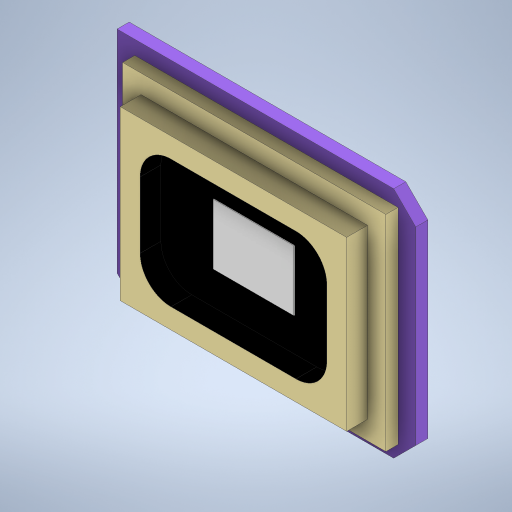
# Autodesk Inventor part: DLP
Saved by Autodesk Inventor 2024 (Build 280153000, 153)
## iProperties
Created: 2024-09-23
Part Number: DLP
Material: Generic
Document SubType Name: Modeling
Designer: PC
Density: 1 g/cm^3
Appearance: Default
Author: PC
Autodesk Inventor part; units mm, degrees
ref_plane "YZ Plane" through (0, 0, 0) normal (1, 0, 0) x (0, 1, 0)
ref_plane "XZ Plane" through (0, 0, 0) normal (0, 1, 0) x (-1, 0, 0)
ref_plane "XY Plane" through (0, 0, 0) normal (0, 0, 1) x (1, 0, 0)
sketch "Sketch1" plane through (0, 0, 0) normal (0, 0, 1) x (1, 0, 0)
  line L0 (3, 0) -> (40.64, 0)
  line L1 (37.64, 31.75) -> (0, 31.75)
  line L2 (0, 31.75) -> (0, 3)
  line L3 (37.64, 31.75) -> (40.64, 28.75)
  line L4 (3, 0) -> (0, 3)
  line L5 (40.64, 3) -> (37.64, 0)
  line L6 (40.64, 28.75) -> (40.64, 3)
  point P0 (0, 0)
  dimension "d4" = 3
  dimension "d5" = 45
  dimension "d6" = 45
  dimension "d7" = 3
  dimension "d8" = 31.75
  dimension "d9" = 40.64
  dimension "d10" = 3
  constraints: 14 end point, 10 coincident, 3 point on line, 1 horizontal, 1 parallel, 1 perpendicular, 1 vertical
  measures "d4" horizontal distance of L5.end L5.start
  measures "d5" angle of L0 L5
  measures "d6" angle of L1 L3
  measures "d7" horizontal distance of L0.start L2.end
  measures "d8" vertical distance of L0.start L1.end
  measures "d9" distance between parallel lines of L2 L6
  measures "d10" horizontal distance of L3.end L1.start
extrude "Extrusion1" add sketch "Sketch1" along normal blind 1.651
sketch "Sketch2" plane through (0, 0, 1.651) normal (0, 0, 1) x (1, 0, 0)
  line L0 (2.413, 29.845) -> (38.227, 29.845)
  line L1 (38.227, 29.845) -> (38.227, 1.905)
  line L2 (38.227, 1.905) -> (2.413, 1.905)
  line L3 (2.413, 1.905) -> (2.413, 29.845)
  line L4 (0, 31.75) -> (0, 3) projected
  line L5 (3, 0) -> (37.64, 0) projected
  line L6 (40.64, 3) -> (40.64, 28.75) projected
  point P0 (0, 0)
  point P1 (0, 17.375)
  point P2 (20.32, 1.905)
  point P3 (20.32, 0)
  point P4 (38.227, 15.875)
  point P5 (40.64, 15.875)
  dimension "d13" = 27.94
  dimension "d14" = 35.814
  constraints: 8 end point, 5 midpoint, 2 parallel, 1 horizontal, 1 horizontal alignment, 1 perpendicular, 1 vertical alignment
  measures "d13" distance of L2.end L0.start
  measures "d14" distance of L1.end L2.end
extrude "Extrusion2" add sketch "Sketch2" along normal blind 1.65
sketch "Sketch3" plane through (0, 0, 3.301) normal (0, 0, 1) x (1, 0, 0)
  line L0 (4.92, 27.305) -> (35.72, 27.305)
  line L1 (35.72, 27.305) -> (35.72, 4.445)
  line L2 (35.72, 4.445) -> (4.92, 4.445)
  line L3 (4.92, 4.445) -> (4.92, 27.305)
  line L4 (2.413, 29.845) -> (2.413, 1.905) projected
  line L5 (3, 0) -> (37.64, 0) projected
  point P0 (0, 0)
  point P1 (4.92, 15.875)
  point P2 (2.413, 15.875)
  point P3 (20.32, 4.445)
  point P4 (20.32, 0)
  dimension "d17" = 22.86
  dimension "d18" = 30.8
  constraints: 8 end point, 4 midpoint, 2 parallel, 1 horizontal, 1 horizontal alignment, 1 perpendicular, 1 vertical alignment
  measures "d17" distance between parallel lines of L2 L0
  measures "d18" distance of L1.end L2.end
extrude "Extrusion3" add sketch "Sketch3" along normal blind 2.83
sketch "Sketch4" plane through (0, 0, 6.131) normal (0, 0, 1) x (1, 0, 0)
  line L0 (11.82, 24.575) -> (28.82, 24.575)
  line L1 (33.02, 20.375) -> (33.02, 11.375)
  line L2 (28.82, 7.175) -> (11.82, 7.175)
  line L3 (7.62, 11.375) -> (7.62, 20.375)
  line L4 (4.92, 27.305) -> (4.92, 4.445) projected
  line L5 (2.413, 1.905) -> (38.227, 1.905) projected
  arc A0 (7.62, 11.375) -> (11.82, 7.175) centre (11.82, 11.375) ccw
  arc A1 (11.82, 24.575) -> (7.62, 20.375) centre (11.82, 20.375) ccw
  arc A2 (33.02, 20.375) -> (28.82, 24.575) centre (28.82, 20.375) ccw
  arc A3 (28.82, 7.175) -> (33.02, 11.375) centre (28.82, 11.375) ccw
  point P0 (0, 0)
  point P1 (7.62, 24.575)
  point P2 (33.02, 7.175)
  point P3 (7.62, 7.175)
  point P4 (7.62, 15.875)
  point P5 (4.92, 15.875)
  point P6 (20.32, 7.175)
  point P7 (20.32, 1.905)
  dimension "d21" = 17.4
  dimension "d22" = 25.4
  dimension "d23" = 4.2
  constraints: 8 end point, 8 point on circle, 8 tangent, 6 point on line, 4 centre point, 4 midpoint, 3 equal radius, 2 parallel, 1 horizontal, 1 horizontal alignment, 1 perpendicular, 1 vertical alignment
  measures "d21" distance of point (7.62, 7.175) point (7.62, 24.575)
  measures "d22" distance of point (33.02, 7.175) point (7.62, 7.175)
  measures "d23" radius of A0
extrude "Extrusion4" cut sketch "Sketch4" against normal blind 2.83
sketch "Sketch5" plane through (0, 0, 3.301) normal (0, 0, 1) x (1, 0, 0)
  line L0 (25.82, 11.75) -> (14.82, 11.75)
  line L1 (14.82, 11.75) -> (14.82, 20)
  line L2 (14.82, 20) -> (25.82, 20)
  line L3 (25.82, 20) -> (25.82, 11.75)
  line L4 (7.62, 11.375) -> (7.62, 20.375) projected
  line L5 (28.82, 7.175) -> (11.82, 7.175) projected
  point P0 (0, 0)
  point P1 (14.82, 15.875)
  point P2 (7.62, 15.875)
  point P3 (20.32, 11.75)
  point P4 (20.32, 7.175)
  dimension "d26" = 11
  dimension "d27" = 8.25
  constraints: 8 end point, 4 midpoint, 2 parallel, 1 horizontal, 1 horizontal alignment, 1 perpendicular, 1 vertical alignment
  measures "d26" distance between parallel lines of L1 L3
  measures "d27" distance of L0.end L1.end
extrude "Extrusion5" add sketch "Sketch5" along normal blind 0.1
body "Solid1"
